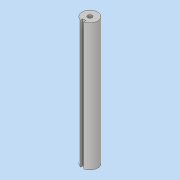
# Autodesk Inventor part: 00_Battery_AAA_Attrap
Saved by Autodesk Inventor 2019.4 (Build 234330000, 330)
## iProperties
Created: 2020-12-03
Part Number: 00_Battery_AAA_Attrap
Material: Generic
Document SubType Name: Modeling
Designer: diederichbenedict
Density: 1 g/cm^3
Appearance: Default
Author: diederichbenedict
Autodesk Inventor part; units mm, degrees
ref_plane "YZ Plane" through (0, 0, 0) normal (1, 0, 0) x (0, 1, 0)
ref_plane "XZ Plane" through (0, 0, 0) normal (0, 1, 0) x (-1, 0, 0)
ref_plane "XY Plane" through (0, 0, 0) normal (0, 0, 1) x (1, 0, 0)
sketch "Sketch1" plane through (0, 0, 0) normal (0, 1, 0) x (-1, 0, 0)
  circle A0 centre (0, 0) radius 5.2
  line L0 (1, 6.7) -> (-1, 6.7)
  line L1 (-1, 6.7) -> (-1, 3.7)
  line L2 (-1, 3.7) -> (1, 3.7)
  line L3 (1, 3.7) -> (1, 6.7)
  line L4 (1, 6.7) -> (-1, 3.7) construction
  line L5 (-1, 6.7) -> (1, 3.7) construction
  point P0 (0, 5.2)
  point P1 (1, 5.1029)
  point P2 (-1, 5.1029)
  dimension "d0" = 10.4
  dimension "d1" = 2
  dimension "d2" = 3
  constraints: 12 end point, 3 point on circle, 2 midpoint, 2 parallel, 2 point on line, 1 centre point, 1 coincident, 1 horizontal, 1 perpendicular
  measures "d0" diameter of A0
  measures "d1" distance of L2.end L1.end
  measures "d2" distance of L1.end L0.end
extrude "Extrusion1" add sketch "Sketch1" along normal blind 84.6 contours A0 L1 L2 L3 picked at (-0.1628, 0.741)
sketch "Sketch2" plane through (0, 84.6, 0) normal (0, 1, 0) x (1, 0, 0)
  circle A0 centre (0, 0) radius 1.45
  dimension "d5" = 2.9
  constraints: 1 centre point, 1 coincident
  measures "d5" diameter of A0
extrude "Extrusion2" cut sketch "Sketch2" against normal blind 20
sketch "Sketch3" plane through (0, 0, 0) normal (0, -1, 0) x (1, 0, 0)
  circle A0 centre (0, 0) radius 1.45 projected
extrude "Extrusion3" cut sketch "Sketch3" against normal blind 20
body "Solid1"
